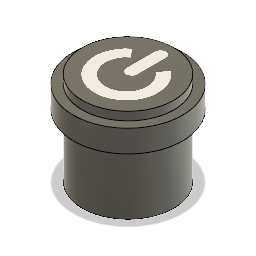
3104 3105 Mini Illuminated Momentary Pushbutton (Autodesk Fusion 360 design; units mm, degrees)
Autodesk Fusion 360 part; units mm, degrees
sketch "Sketch1" plane through (0, 0, 0) normal (0, 1, 0) x (1, 0, 0)
  circle A0 centre (0, 0) radius 4.1
  dimension "d2" = 8.2
  measures "d2" diameter of A0
extrude "Extrude1" add sketch "Sketch1" along normal blind 8.4
sketch "Sketch2" plane through (0, 8.4, 0) normal (0, 1, 0) x (-1, 0, 0)
  circle A0 centre (0, 0) radius 4.1
  circle A1 centre (0, 0) radius 4.9
  dimension "d5" = 9.8
  measures "d5" diameter of A1
extrude "Extrude2" add sketch "Sketch2" against normal blind 2 from surface at -0.75
equation "d6 = -ActuatorDepth"
equation "ActuatorDepth = 0.75 mm" comment "Not in the drawing, so this is eyeballed"
